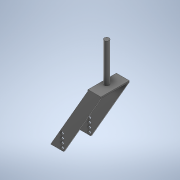
# Autodesk Inventor part: Wheel-Housing
Saved by Autodesk Inventor 2022 (Build 260153000, 153)
## iProperties
Created: 2021-12-05
Part Number: Wheel-Housing
Material: Generic
Document SubType Name: Modeling
Designer: Vedic
Density: 1 g/cm^3
Appearance: Default
Author: Vedic
Autodesk Inventor part; units mm, degrees
ref_plane "YZ Plane" through (0, 0, 0) normal (1, 0, 0) x (0, 1, 0)
ref_plane "XZ Plane" through (0, 0, 0) normal (0, 1, 0) x (-1, 0, 0)
ref_plane "XY Plane" through (0, 0, 0) normal (0, 0, 1) x (1, 0, 0)
sketch "Sketch1" plane through (0, 0, 0) normal (0, 1, 0) x (-1, 0, 0)
  line L0 (18.2162, 26.4548) -> (-7.1838, 26.4548)
  line L1 (-7.1838, 26.4548) -> (-7.1838, -24.3452)
  line L2 (-7.1838, -24.3452) -> (18.2162, -24.3452)
  line L3 (18.2162, -24.3452) -> (18.2162, 26.4548)
  point P0 (0, 0)
  dimension "d0" = 50.8
  dimension "d1" = 25.4
  constraints: 8 end point, 2 parallel, 1 horizontal, 1 perpendicular
  measures "d0" distance of L2.end L0.start
  measures "d1" distance of L1.end L2.end
extrude "Extrusion1" add sketch "Sketch1" along normal blind 2.54
sketch "Sketch2" plane through (7.1838, 0, -24.3452) normal (0, 0, -1) x (-1, 0, 0)
  line L0 (0, 0) -> (73.3235, -127)
  line L1 (73.3235, -127) -> (98.7235, -127)
  line L2 (0, 0) -> (25.4, 0) projected
  line L3 (98.7235, -127) -> (25.4, 0)
  line L4 (0, 2.54) -> (25.4, 2.54) projected
  line L5 (0, 0) -> (0, 2.54)
  line L6 (0, 2.54) -> (25.4, 2.54)
  line L7 (25.4, 2.54) -> (25.4, 0)
  point P0 (7.1838, 0)
  dimension "d4" = 60
  dimension "d5" = 127
  constraints: 12 end point, 2 equal length, 2 perpendicular, 1 horizontal
  measures "d4" angle of L2 L0
  measures "d5" distance between parallel lines of L2 L1
extrude "Extrusion2" add sketch "Sketch2" along normal blind 2.54
sketch "Sketch3" plane through (-18.2162, 0, 26.4548) normal (0, 0, 1) x (1, 0, 0)
  line L0 (0, 0) -> (0, 2.54) projected
  line L1 (0, 0) -> (0, 2.54)
  line L2 (25.4, 0) -> (25.4, 2.54) projected
  line L3 (0, 2.54) -> (25.4, 2.54)
  line L4 (25.4, 2.54) -> (25.4, 0)
  line L5 (25.4, 0) -> (-47.9235, -127) projected
  line L6 (25.4, 0) -> (-47.9235, -127)
  line L7 (-47.9235, -127) -> (-73.3235, -127) projected
  line L8 (-47.9235, -127) -> (-73.3235, -127)
  line L9 (-73.3235, -127) -> (0, 0)
  point P0 (18.2162, 0)
  constraints: 12 end point, 4 equal length, 2 perpendicular
extrude "Extrusion3" add sketch "Sketch3" along normal blind 2.54
sketch "Sketch4" plane through (0, 2.54, 0) normal (0, 1, 0) x (1, 0, 0)
  line L0 (7.1838, -26.4548) -> (7.1838, 24.3452) construction
  line L1 (-66.1396, -28.9948) -> (7.1838, -28.9948) construction
  line L2 (7.1838, -1.0548) -> (-9.3262, -1.0548) construction
  line L3 (-9.3262, -1.0548) -> (-9.3262, -28.9948) construction
  line L4 (-9.3262, -28.9948) -> (7.1838, -28.9948) construction
  line L5 (7.1838, -28.9948) -> (7.1838, -1.0548) construction
  circle A0 centre (-9.3262, -1.0548) radius 4.7625
  dimension "d11" = 16.51
  dimension "d12" = 9.525
  constraints: 8 end point, 2 parallel, 1 centre point, 1 coincident, 1 horizontal, 1 midpoint, 1 perpendicular, 1 point on line
  measures "d11" distance between parallel lines of L0 L3
  measures "d12" diameter of A0
extrude "Extrusion4" add sketch "Sketch4" along normal blind 76.2
sketch "Sketch5" plane through (7.1838, 0, -26.8852) normal (0, 0, -1) x (-1, 0, 0)
  line L0 (98.7235, -127) -> (25.4, 0) projected
  line L1 (98.7235, -127) -> (75.8635, -127)
  line L2 (75.8635, -127) -> (75.8635, -87.4053)
  line L3 (75.8635, -87.4053) -> (98.7235, -87.4053)
  line L4 (98.7235, -87.4053) -> (98.7235, -127)
  circle A0 centre (75.8635, -122.2375) radius 3.175
  circle A1 centre (75.8635, -113.9825) radius 3.175
  circle A2 centre (75.8635, -105.7275) radius 3.175
  circle A3 centre (75.8635, -97.4725) radius 3.175
  point P0 (7.1838, 0)
  dimension "d15" = 6.35
  dimension "d16" = 4.7625
  dimension "d17" = 22.86
  dimension "d20" = 8.255
  constraints: 8 end point, 4 centre point, 2 parallel, 2 point on line, 1 horizontal, 1 perpendicular, 1 vertical, 6 other
  measures "d15" diameter of A0
  measures "d16" distance from line of L1 A0.centre
  measures "d17" distance of L2.end L3.end
  measures "d20" distance of A0.centre A1.centre
extrude "Extrusion5" cut sketch "Sketch5" against normal through all contours A3 L2 | L2 A3 | A0 L2 | L2 A0 | A2 L2 | L2 A2 | A1 L2 | L2 A1
sketch "Sketch6" plane through (-18.2162, 0, 28.9948) normal (0, 0, 1) x (1, 0, 0)
  circle A0 centre (-50.4635, -105.7275) radius 3.175 projected
  circle A1 centre (-50.4635, -105.7275) radius 101.6 construction
  line L0 (25.4, 2.54) -> (0, 2.54) projected
  point P0 (18.2162, 0)
  point P1 (-50.4635, -4.1275)
  dimension "d27" = 203.2
  dimension "d28" = 6.6675
  constraints: 1 coincident, 1 vertical alignment, 2 other
  measures "d28" distance from line of L0 point (-50.463, -4.127)
body "Solid1"
